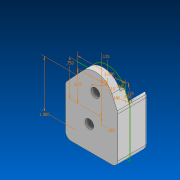
# Autodesk Inventor part: Elevator Tensioner
Saved by Autodesk Inventor 2022 (Build 260153000, 153)
## iProperties
Created: 2022-04-08
Part Number: Elevator Tensioner
Material: Generic
Document SubType Name: Modeling
Designer: score_nygvs6w
Density: 1 g/cm^3
Appearance: Default
Author: score_nygvs6w
Autodesk Inventor part; units mm, degrees
ref_plane "YZ Plane" through (0, 0, 0) normal (1, 0, 0) x (0, 1, 0)
ref_plane "XZ Plane" through (0, 0, 0) normal (0, 1, 0) x (-1, 0, 0)
ref_plane "XY Plane" through (0, 0, 0) normal (0, 0, 1) x (1, 0, 0)
sketch "Sketch1" plane through (0, 0, 0) normal (0, 0, 1) x (1, 0, 0)
  line L0 (12.7, -12.7) -> (-12.7, -12.7)
  line L1 (-12.7, -12.7) -> (-12.7, 12.7)
  line L2 (-12.7, 12.7) -> (12.7, 12.7)
  line L3 (12.7, 12.7) -> (12.7, -12.7)
  line L4 (12.7, -12.7) -> (-12.7, 12.7) construction
  line L5 (-12.7, -12.7) -> (12.7, 12.7) construction
  circle A0 centre (3.175, 15.875) radius 9.525
  line L6 (12.7, 12.7) -> (14.986, 12.7)
  line L7 (14.986, 12.7) -> (14.986, -12.7)
  line L8 (14.986, -12.7) -> (12.7, -12.7)
  line L9 (12.7, -12.7) -> (12.7, 12.7) construction
  line L10 (-1.6186, 14.8001) -> (-0.1527, 19.489) construction
  line L11 (-0.1527, 19.489) -> (4.6409, 20.5639) construction
  line L12 (4.6409, 20.5639) -> (7.9686, 16.9499) construction
  line L13 (7.9686, 16.9499) -> (6.5027, 12.261) construction
  line L14 (6.5027, 12.261) -> (1.7091, 11.1861) construction
  line L15 (1.7091, 11.1861) -> (-1.6186, 14.8001) construction
  circle A1 centre (3.175, 15.875) radius 2.286
  circle A2 centre (3.175, 15.875) radius 4.0005
  circle A3 centre (0, 0) radius 2.286
  line L16 (-12.7, 12.7) -> (-3.8307, 22.3284)
  line L17 (14.986, 12.7) -> (11.8898, 19.7191)
  line L18 (12.7, 12.7) -> (12.7, 15.875)
  line L19 (12.7, 15.875) -> (12.7, 17.8824)
  line L20 (-12.7, 19.05) -> (12.7, 19.05)
  point P0 (14.986, 4.9127)
  point P1 (14.986, 2.5046)
  point P2 (14.986, -1.9271)
  point P3 (12.1553, 12.7)
  point P4 (-5.8053, 12.7)
  point P5 (5.6088, 19.05)
  point P6 (12.1553, 19.05)
  point P7 (-6.8506, 19.05)
  point P8 (0.7412, 19.05)
  point P9 (12.185, 19.05)
  dimension "d0" = 25.4
  dimension "d1" = 25.4
  dimension "d3" = 19.05
  dimension "d5" = 8.509
  dimension "d6" = 4.572
  dimension "d13" = 8.001
  dimension "d17" = 4.572
  dimension "d19" = 2.286
  dimension "d20" = 15.875
  dimension "d21" = 3.175
  dimension "d22" = 19.05
  constraints: 42 end point, 4 centre point, 4 coincident, 4 parallel, 4 point on line, 3 horizontal, 3 midpoint, 3 point on circle, 3 tangent, 2 perpendicular, 1 collinear, 13 other
  measures "d0" distance between parallel lines of L3 L1
  measures "d1" distance between parallel lines of L0 L2
  measures "d3" diameter of A0
  measures "d5" distance between parallel lines of L11 L14
  measures "d6" diameter of A1
  measures "d13" diameter of A2
  measures "d17" diameter of A3
  measures "d19" distance between parallel lines of L3 L7
  measures "d20" vertical distance of A0.centre point (0, 0)
  measures "d21" horizontal distance of point (0, 0) A0.centre
  measures "d22" distance from line of L20 point (0, 0)
extrude "Extrusion1" add sketch "Sketch1" along normal blind 6.35
extrude "Extrusion2" add sketch "Sketch1" against normal blind 9.525 contours L3 L6 L7 L8 | L18 L19 L17 L6
extrude "Extrusion3" cut sketch "Sketch1" along normal blind 2.54 contours A2 L2 | L2 A2 L20 | L20 A2
fillet "Fillet2" radius 3.175 4 edges at (14.986, 12.7, -1.5875) (14.986, -12.7, -1.5875) (-12.7, -12.7, 3.175) (-12.7, 12.7, 3.175)
fillet "Fillet1" radius 1.27 2 edges at (14.986, 1.2529, -9.525) (12.7, 17.8824, -4.7625)
extrude "Extrusion4" cut sketch "Sketch1" along normal blind 2.286 contours L16 A0 L20 | L20 A2 A0 | A0 L17 L20
fillet "Fillet3" radius 1.27 2 edges at (0.7412, 19.05, 1.143) (5.6088, 19.05, 1.143)
body "Solid1"
